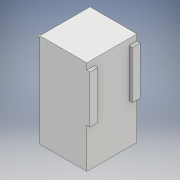
# Autodesk Inventor part: ax12
Saved by Autodesk Inventor 2017 (Build 210142000, 142)
## iProperties
Created: 2017-11-23
Part Number: ax12
Material: ABS Plastic
Document SubType Name: Modeling
Designer: Biscuit
Density: 1.06 g/cm^3
Appearance: Smooth - White
Author: Biscuit
Autodesk Inventor part; units mm, degrees
ref_plane "YZ Plane" through (0, 0, 0) normal (1, 0, 0) x (0, 1, 0)
ref_plane "XZ Plane" through (0, 0, 0) normal (0, 1, 0) x (-1, 0, 0)
ref_plane "XY Plane" through (0, 0, 0) normal (0, 0, 1) x (1, 0, 0)
sketch "Sketch1" plane through (0, 0, 0) normal (0, 1, 0) x (-1, 0, 0)
  line L0 (0, 0) -> (30, 0)
  line L1 (30, 0) -> (30, -60)
  line L2 (30, -60) -> (0, -60)
  line L3 (0, -60) -> (0, 0)
  dimension "d0" = 30
  dimension "d1" = 60
  constraints: 8 end point, 2 parallel, 1 horizontal, 1 perpendicular
  measures "d0" distance of L0.start L0.end
  measures "d1" distance of L0.end L1.end
extrude "Extrusion1" add sketch "Sketch1" along normal blind 32
sketch "Sketch2" plane through (0, 32, 0) normal (0, 1, 0) x (1, 0, 0)
  circle A0 centre (-15, 11) radius 3.5
  line L0 (0, 0) -> (-30, 0) projected
  line L1 (0, 0) -> (0, 60) projected
  dimension "d4" = 7
  dimension "d5" = 11
  dimension "d6" = 30
  dimension "d7" = 15
  constraints: 1 centre point
  measures "d4" diameter of A0
  measures "d5" distance from line of L0 A0.centre
  measures "d6" distance of L0.start L0.end
  measures "d7" distance from line of L1 A0.centre
extrude "Extrusion2" cut sketch "Sketch2" against normal blind 10
sketch "Sketch3" plane through (0, 0, 0) normal (1, 0, 0) x (0, 0, -1)
  line L0 (0, 32) -> (60, 32) projected
  line L1 (4, 32) -> (34.5, 32)
  line L2 (34.5, 32) -> (34.5, 27)
  line L3 (34.5, 27) -> (4, 27)
  line L4 (4, 27) -> (4, 32)
  line L5 (60, 0) -> (0, 0) projected
  line L6 (34.5, 0) -> (4, 0)
  line L7 (4, 0) -> (4, 5)
  line L8 (4, 5) -> (34.5, 5)
  line L9 (34.5, 5) -> (34.5, 0)
  line L10 (0, 0) -> (0, 32) projected
  dimension "d10" = 5
  dimension "d11" = 5
  dimension "d12" = 30.5
  dimension "d13" = 30.5
  dimension "d16" = 4
  constraints: 16 end point, 4 parallel, 4 point on line, 2 horizontal, 2 perpendicular
  measures "d10" distance of L6.end L7.end
  measures "d11" distance of L3.end L1.start
  measures "d12" distance of L2.end L3.end
  measures "d13" distance of L7.end L8.end
  measures "d16" distance between parallel lines of L10 L4
extrude "Extrusion3" add sketch "Sketch3" along normal blind 2
sketch "Sketch4" plane through (-30, 0, -60) normal (-1, 0, 0) x (0, 0, 1)
  point P0 (60, 0)
equation "\"d7\" = 0.5 * d6"
equation "\"d10\" = d11"
body "Solid1"
